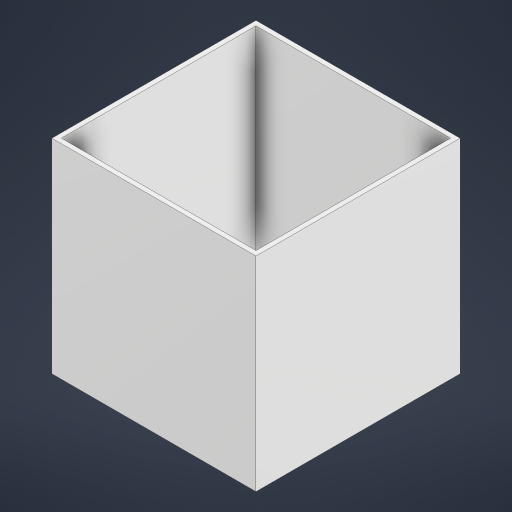
# Autodesk Inventor part: Cube
Saved by Autodesk Inventor 2023 (Build 270158000, 158)
## iProperties
Created: 2023-11-15
Part Number: Cube
Material: ABS Plastic
Document SubType Name: Modeling
Designer: dexter.hedman
Density: 1.06 g/cm^3
Appearance: Smooth - White
Mass: 29.4786 g
Surface Area: 232.78 cm^2
Volume: 27.81 cm^3
Author: dexter.hedman
Autodesk Inventor part; units mm, degrees
ref_plane "YZ Plane" through (0, 0, 0) normal (1, 0, 0) x (0, 1, 0)
ref_plane "XZ Plane" through (0, 0, 0) normal (0, 1, 0) x (-1, 0, 0)
ref_plane "XY Plane" through (0, 0, 0) normal (0, 0, 1) x (1, 0, 0)
sketch "Sketch2" plane through (0, 0, 0) normal (0, 1, 0) x (-1, 0, 0)
  line L0 (27, 27) -> (-27, 27)
  line L1 (-27, 27) -> (-27, -27)
  line L2 (-27, -27) -> (27, -27)
  line L3 (27, -27) -> (27, 27)
  line L4 (27, 27) -> (-27, -27) construction
  line L5 (-27, 27) -> (27, -27) construction
  line L6 (25.75, -25.75) -> (-25.75, -25.75)
  line L7 (-25.75, -25.75) -> (-25.75, 25.75)
  line L8 (-25.75, 25.75) -> (25.75, 25.75)
  line L9 (25.75, 25.75) -> (25.75, -25.75)
  dimension "d31" = 54
  dimension "d32" = 54
  dimension "d43" = 1.25
  constraints: 20 end point, 4 parallel, 2 perpendicular, 1 horizontal, 3 other
  measures "d31" distance of L2.end L1.end
  measures "d32" distance of L1.end L0.end
  measures "d43" distance between parallel lines of L2 L6
extrude "Extrusion5" add sketch "Sketch2" along normal blind 54
body "Solid5"
